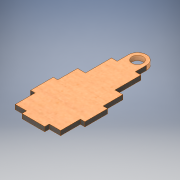
# Autodesk Inventor part: PistonPart3
Saved by Autodesk Inventor 2019 (Build 230136000, 136)
## iProperties
Created: 2021-01-03
Part Number: PistonPart3
Material: Дерево (вишня)
Document SubType Name: Modeling
Designer: Professional
Density: 0.63 g/cm^3
Appearance: Вишневое дерево — натуральный — со слабым глянцем
Author: Professional
Autodesk Inventor part; units mm, degrees
ref_plane "YZ Plane" through (0, 0, 0) normal (1, 0, 0) x (0, 1, 0)
ref_plane "XZ Plane" through (0, 0, 0) normal (0, 1, 0) x (-1, 0, 0)
ref_plane "XY Plane" through (0, 0, 0) normal (0, 0, 1) x (1, 0, 0)
sketch "Эскиз1" plane through (0, 0, 0) normal (0, 1, 0) x (-1, 0, 0)
  line L0 (0, 0) -> (8, 0) construction
  line L1 (8, 0) -> (8, 4)
  line L2 (8, 4) -> (13, 4)
  line L3 (13, 4) -> (13, 27)
  line L4 (13, 27) -> (20, 27)
  line L5 (0, 0) -> (0, 86)
  line L6 (0, 0) -> (-8, 0) construction
  line L7 (-8, 0) -> (-8, 4)
  line L8 (-8, 4) -> (-13, 4)
  line L9 (-13, 4) -> (-13, 27)
  line L10 (-13, 27) -> (-20, 27)
  line L11 (20, 27) -> (20, 44.5)
  line L12 (20, 44.5) -> (24, 44.5)
  line L13 (24, 44.5) -> (24, 64.5)
  line L14 (24, 64.5) -> (20, 64.5)
  line L15 (-20, 27) -> (-20, 44.5)
  line L16 (-20, 44.5) -> (-24, 44.5)
  line L17 (-24, 44.5) -> (-24, 64.5)
  line L18 (-24, 64.5) -> (-20, 64.5)
  line L19 (20, 64.5) -> (20, 82)
  line L20 (20, 82) -> (10, 82)
  line L21 (10, 82) -> (10, 86)
  line L22 (10, 86) -> (0, 86)
  line L23 (-20, 64.5) -> (-20, 82)
  line L24 (-20, 82) -> (-10, 82)
  line L25 (-10, 82) -> (-10, 86)
  line L26 (-10, 86) -> (0, 86)
  line L27 (-8, 0) -> (-8, -6)
  line L28 (8, -6) -> (8, 0)
  arc A0 (-8, -6) -> (8, -6) centre (0, -6) ccw
  circle A1 centre (0, -6) radius 5
  dimension "d0" = 16
  dimension "d1" = 26
  dimension "d2" = 40
  dimension "d3" = 4
  dimension "d4" = 23
  dimension "d5" = 55
  dimension "d6" = 20
  dimension "d7" = 20
  dimension "d10" = 6
  dimension "d11" = 10
  constraints: 59 end point, 12 symmetric about line, 9 perpendicular, 5 vertical, 3 equal length, 2 centre point, 2 point on circle, 2 tangent, 1 coincident, 1 horizontal, 1 vertical alignment
  measures "d0" distance between parallel lines of L1 L7
  measures "d1" distance between parallel lines of L9 L3
  measures "d2" distance between parallel lines of L15 L11
  measures "d3" distance of L11.end L12.end
  measures "d4" distance of L2.end L3.end
  measures "d5" distance between parallel lines of L20 L4
  measures "d6" distance between parallel lines of L14 L12
  measures "d7" distance between parallel lines of L25 L21
  measures "d10" distance of A0.centre L0.start
  measures "d11" diameter of A1
extrude "Выдавливание1" add sketch "Эскиз1" along normal blind 4
